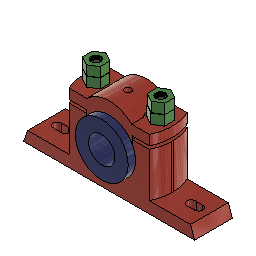
plumber block 3d (Autodesk Fusion 360 design; units mm, degrees)
Autodesk Fusion 360 part; units mm, degrees
sketch "Sketch1" plane through (0, 0, 0) normal (0, 1, 0) x (1, 0, 0)
  line L0 (23.6292, -4.2078) -> (27.987, -4.2078)
  line L1 (27.987, -4.2078) -> (27.987, -20.2078)
  line L2 (27.987, -20.2078) -> (53.987, -20.2078)
  line L3 (53.987, -20.2078) -> (53.987, 33.7922)
  line L4 (53.987, 33.7922) -> (98.9042, 33.7922)
  line L5 (103.9042, 47.7922) -> (-0.0958, 47.7922)
  line L6 (-0.0958, 47.7922) -> (-0.0958, 24.0008)
  line L7 (98.9042, 33.7922) -> (103.9042, 47.7922)
  arc A0 (23.6292, -4.2078) -> (-0.0958, 24.0008) centre (0, 0) ccw
  line L8 (-54.1786, 33.7922) -> (-99.0958, 33.7922)
  line L9 (-99.0958, 33.7922) -> (-104.0958, 47.7922)
  line L10 (-104.0958, 47.7922) -> (-0.0958, 47.7922)
  arc A1 (-0.0958, 24.0008) -> (-23.8208, -4.2078) centre (-0.1916, 0) ccw
  line L11 (-28.1786, -4.2078) -> (-28.1786, -20.2078)
  line L12 (-28.1786, -20.2078) -> (-54.1786, -20.2078)
  line L13 (-54.1786, -20.2078) -> (-54.1786, 33.7922)
  line L14 (-23.8208, -4.2078) -> (-28.1786, -4.2078)
  point P0 (-0.1916, 0)
  dimension "d3" = 26
  dimension "d5" = 16
  dimension "d6" = 104
  dimension "d7" = 5
  dimension "d39" = 68
  dimension "d61" = 44.9172
  dimension "d62" = 14
  constraint coincident A0.centre origin
  constraint perpendicular L0 L1
  constraint perpendicular L1 L2
  constraint perpendicular L2 L3
  constraint perpendicular L3 L4
  constraint perpendicular L5 L6
  constraint symmetric A0.centre L6 A1.centre
  constraint symmetric L0.end L6 L11.start
  constraint symmetric L1.end L6 L11.end
  constraint symmetric L2.end L6 L12.end
  constraint symmetric L3.end L6 L8.start
  constraint symmetric L4.end L6 L8.end
  constraint symmetric L5.start L6 L9.end
  constraint symmetric L5.end L6 L10.end
  constraint symmetric L6 A0.end A1.start
  constraint symmetric L6 L0.start A1.end
  constraint symmetric L6 A0 A1
  constraint horizontal L4
  constraint horizontal L5
  measures "d3" distance of L1.end L2.end
  measures "d5" distance of L0.end L1.end
  measures "d6" distance of L5.start L5.end
  measures "d7" horizontal distance of L4.end L5.start
  measures "d39" distance of L2.end L5
  measures "d61" distance of L3.end L4.end
  measures "d62" distance of L4 L5
extrude "Extrude1" add sketch "Sketch1" along normal mid plane 46 makes body 1
sketch "Sketch2" plane through (0, 0, 0) normal (0, 1, 0) x (1, 0, 0)
  line L0 (0, 0) -> (0, -8)
  line L1 (0, -8) -> (28, -8)
  line L2 (28, -8) -> (28, -24)
  line L3 (28, -24) -> (54, -24)
  line L4 (54, -24) -> (54, -36)
  line L5 (54, -36) -> (27.1477, -36)
  line L6 (-28, -24) -> (-54, -24)
  line L7 (-54, -36) -> (-27.1477, -36)
  line L8 (-28, -8) -> (-28, -24)
  line L9 (-54, -24) -> (-54, -36)
  line L10 (0, -8) -> (-28, -8)
  arc A0 (-22.6274, -8) -> (22.6274, -8) centre (0, 0) ccw
  arc A1 (-27.1477, -36) -> (27.1477, -36) centre (0, -8) ccw
  dimension "d11" = 8
  dimension "d12" = 28
  dimension "d13" = 16
  dimension "d14" = 26
  dimension "d15" = 12
  dimension "d64" = 48
  dimension "d65" = 78
  constraint coincident L0.start A0.centre
  constraint vertical L0
  constraint perpendicular L0 L1
  constraint perpendicular L1 L2
  constraint perpendicular L2 L3
  constraint perpendicular L1 L4
  constraint perpendicular L4 L5
  constraint coincident L1 A0.end
  constraint coincident L10 A0.start
  constraint coincident L0.end L1.start
  constraint horizontal L7
  measures "d11" distance of L0.start L0.end
  measures "d12" distance of L0.end L1.end
  measures "d13" distance of L1.end L2.end
  measures "d14" distance of L2.end L3.end
  measures "d15" distance of L3.end L4.end
  measures "d64" diameter of A0
  measures "d65" diameter of A1
extrude "Extrude2" add sketch "Sketch2" along normal mid plane 46 separate body contours L1 L2 L3 L4 L5 L6 L7 L8 L9 L10 A0 A1 makes body 2
sketch "Sketch3" plane through (0, 0, -47.7922) normal (0, 0, -1) x (1, 0, 0)
  line L0 (-104.0958, 23) -> (-104.0958, -23)
  line L1 (-104.0958, -23) -> (103.9042, -23)
  line L2 (103.9042, -23) -> (103.9042, 23)
  line L3 (103.9042, 23) -> (-104.0958, 23)
  circle A0 centre (0, 0) radius 4
  circle A1 centre (0, 0) radius 54
  circle A2 centre (0, 0) radius 83.1695
  circle A3 centre (38.9975, 0.4423) radius 7
  line L4 (51.9975, -12.5577) -> (25.9975, -12.5577)
  line L5 (25.9975, -12.5577) -> (25.9975, 13.4423)
  line L6 (25.9975, 13.4423) -> (51.9975, 13.4423)
  line L7 (51.9975, 13.4423) -> (51.9975, -12.5577)
  line L8 (51.9975, -12.5577) -> (25.9975, 13.4423) construction
  line L9 (25.9975, -12.5577) -> (51.9975, 13.4423) construction
  line L10 (0, 0) -> (-0.0958, 23)
  arc A4 (-78.3843, -5.3343) -> (-78.4652, 4.6223) centre (-77, -0.3444) ccw
  arc A5 (-86.4872, 4.5537) -> (-86.4043, -5.3996) centre (-86.4457, -0.4229) ccw
  line L11 (-51.8911, -12.9904) -> (-26.1085, 13.2253) construction
  line L12 (-25.892, -12.7738) -> (-52.1076, 13.0087) construction
  line L13 (-51.8911, -12.9904) -> (-25.892, -12.7738)
  line L14 (-78.3843, -5.3343) -> (-86.4043, -5.3996)
  line L15 (-86.4872, 4.5537) -> (-78.4652, 4.6223)
  line L16 (-25.892, -12.7738) -> (-26.1085, 13.2253)
  circle A6 centre (-38.9998, 0.1175) radius 7
  line L17 (-26.1085, 13.2253) -> (-52.1076, 13.0087)
  line L18 (-86.4457, -0.4229) -> (-77, -0.3444) construction
  line L19 (-52.1076, 13.0087) -> (-51.8911, -12.9904)
  line L20 (78.426, -4.6813) -> (86.4463, -4.6797)
  arc A7 (78.424, 5.2757) -> (78.426, -4.6813) centre (77.0002, 0.2969) ccw
  line L21 (86.4463, 0.2971) -> (77.0002, 0.2969) construction
  line L22 (86.4463, 5.2739) -> (78.424, 5.2757)
  arc A8 (86.4463, -4.6797) -> (86.4463, 5.2739) centre (86.4463, 0.2971) ccw
  point P0 (38.9975, 0.4423)
  point P1 (-38.9998, 0.1175)
  dimension "d20" = 8
  dimension "d21" = 108
  dimension "d22" = 14
  dimension "d23" = 26
  dimension "d24" = 26
  dimension "d27" = 39
  dimension "d63" = 77
  constraint coincident A0.centre A1.centre
  constraint concentric A0 A2
  constraint horizontal L4
  constraint perpendicular L4 L5
  constraint parallel L4 L6
  constraint parallel L5 L7
  constraint coincident L8 P0
  constraint coincident L9 P0
  constraint coincident P0 A3.centre
  constraint midpoint L3 L10.end
  constraint symmetric A3 L10 A6
  constraint symmetric L4.start L10 L11.start
  constraint symmetric L4.end L10 L12.start
  constraint symmetric L5.end L10 L11.end
  constraint symmetric L6.end L10 L12.end
  constraint symmetric P0 L10 P1
  constraint symmetric L10 A5.start L22.start
  constraint symmetric L10 A4.end A7.start
  constraint symmetric L10 A5.end L20.end
  constraint symmetric L10 A4.start L20.start
  constraint symmetric L10 A4 A7
  constraint symmetric L10 A5 A8
  measures "d20" diameter of A0
  measures "d21" diameter of A1
  measures "d22" diameter of A3
  measures "d23" distance of L5.end L6.end
  measures "d24" distance of L4.end L5.end
  measures "d27" distance of A0.centre P0
  measures "d63" horizontal distance of A0.centre A4.centre
extrude "Extrude3" cut sketch "Sketch3" against normal blind 80 from surface at -14 contours L1 L3 A1 A2 A4 L14 L15 | L1 L3 A1 A2 L20 A7 L22 | A2 A4 L14 L15 | A2 A5 L14 L15 bodies 1 2
extrude "Extrude4" cut sketch "Sketch3" against normal blind 120 contours A2 A4 L14 L15 | A2 A5 L14 L15 | A2 L20 L22 A8 | A2 L20 A7 L22 | A3 | A6 bodies 1 2
extrude "Extrude5" cut sketch "Sketch3" against normal blind 10 contours L4 L5 L6 L7 | L13 L16 L17 L19 bodies 1
extrude "Extrude8" cut sketch "Sketch3" against normal blind 25 contours A0 bodies 1
sketch "Sketch4" plane through (0, 0, 0) normal (1, 0, 0) x (0, 1, 0)
  line L0 (0, 0) -> (32, 0)
  line L1 (32, 0) -> (32, 32)
  line L2 (32, 32) -> (23, 32)
  line L3 (23, 32) -> (23, 24)
  line L4 (23, 24) -> (14, 24)
  line L5 (14, 24) -> (14, 22)
  line L6 (14, 22) -> (0, 22)
  line L7 (0, 22) -> (0, 0)
  line L8 (0, 16) -> (32, 16)
  line L9 (0, 0) -> (-32, 0)
  line L10 (0, 16) -> (-32, 16)
  line L11 (-14, 22) -> (0, 22)
  line L12 (-23, 32) -> (-23, 24)
  line L13 (-32, 32) -> (-23, 32)
  line L14 (-32, 0) -> (-32, 32)
  line L15 (-23, 24) -> (-14, 24)
  line L16 (-14, 24) -> (-14, 22)
  dimension "d43" = 32
  dimension "d44" = 32
  dimension "d45" = 23
  dimension "d46" = 14
  dimension "d47" = 24
  dimension "d48" = 22
  dimension "d49" = 16
  constraint coincident L0.start L7.end
  constraint horizontal L0
  constraint perpendicular L0 L1
  constraint perpendicular L1 L2
  constraint perpendicular L2 L3
  constraint perpendicular L3 L4
  constraint perpendicular L4 L5
  constraint perpendicular L5 L6
  constraint perpendicular L7 L8
  constraint symmetric L0.start L7 L9.start
  constraint symmetric L0.end L7 L9.end
  constraint symmetric L1.end L7 L13.start
  constraint symmetric L2.end L7 L12.start
  constraint symmetric L3.end L7 L12.end
  constraint symmetric L4.end L7 L15.end
  constraint symmetric L5.end L7 L11.start
  constraint symmetric L6.end L7 L11.end
  constraint symmetric L7 L8.end L10.end
  constraint midpoint L1 L8.end
  measures "d43" distance of L0.start L0.end
  measures "d44" distance of L0.end L1.end
  measures "d45" distance of L2.end L7
  measures "d46" distance of L5 L6.end
  measures "d47" distance of L0 L4
  measures "d48" distance of L0 L6
  measures "d49" vertical distance of L0.start L8.start
revolve "Revolve1" add sketch "Sketch4" angle 360 about axis through (0, 0, 0) along (0, 1, 0) separate body contours L7 L10 L11 L12 L13 L14 L15 L16 | L1 L2 L3 L4 L5 L6 L7 L8 makes body 3
extrude "Extrude7" add sketch "Sketch3" along normal blind 9 from surface at -27 contours A0 bodies 3
ref_plane "WorkPlane2" through (0, -5.0102, 47) normal (0, 0, 1) x (-1, 0, 0)
sketch "Sketch6" plane through (0, 0, 47) normal (0, 0, 1) x (1, 0, 0)
  circle A0 centre (0, 0) radius 4
  circle A1 centre (0, 0) radius 3
  dimension "d67" = 8
  dimension "d68" = 6
  constraint coincident A0.centre A1.centre
  measures "d67" diameter of A0
  measures "d68" diameter of A1
extrude "Extrude9" cut sketch "Sketch6" against normal blind 60 contours A1 bodies 2 3
extrude "Extrude10" cut sketch "Sketch6" against normal blind 16 bodies 2
sketch "Sketch7" plane through (0, 0, -37.7922) normal (0, 0, -1) x (1, 0, 0)
  circle A0 centre (-38.9998, 0.1175) radius 7
  line L0 (-52.1076, 13.0087) -> (-51.8911, -12.9904)
  line L1 (-51.8911, -12.9904) -> (-25.892, -12.7738)
  line L2 (-25.892, -12.7738) -> (-26.1085, 13.2253)
  line L3 (-26.1085, 13.2253) -> (-52.1076, 13.0087)
  circle A1 centre (-38.9998, 0.1175) radius 6
  line L4 (-26.9998, -11.8825) -> (-50.9998, -11.8825)
  line L5 (-50.9998, -11.8825) -> (-50.9998, 12.1175)
  line L6 (-50.9998, 12.1175) -> (-26.9998, 12.1175)
  line L7 (-26.9998, 12.1175) -> (-26.9998, -11.8825)
  line L8 (-26.9998, -11.8825) -> (-50.9998, 12.1175) construction
  line L9 (-50.9998, -11.8825) -> (-26.9998, 12.1175) construction
  point P0 (-38.9998, 0.1175)
  dimension "d75" = 12
  dimension "d76" = 24
  dimension "d77" = 24
  constraint concentric A0 A1
  constraint horizontal L4
  constraint perpendicular L4 L5
  constraint parallel L4 L6
  constraint parallel L5 L7
  constraint coincident L8 P0
  constraint coincident L9 P0
  constraint coincident P0 A0.centre
  measures "d75" diameter of A1
  measures "d76" distance of L5.end L6.end
  measures "d77" distance of L4.start L6.end
extrude "Extrude11" add sketch "Sketch7" along normal blind 8 separate body contours A0 | A1 | L4 L5 L6 L7 makes body 4
extrude "Extrude12" add sketch "Sketch7" against normal blind 95 contours A1 bodies 4
thread "Thread1" "ISO Metric profile 12.0 M12x1.75 6g" major diameter 11.8335 minor diameter 9.8365 pitch 1.75 angle 60 modelled right hand crest width 0.2518 on face at (-33.0073, 0.1816, 25.5412) from (-38.9998, -0.1175, 28.7078) to (-38.9998, -0.1175, 56.7078) crest through (-33.0831, -0.1175, -38.2297) on bodies 4
fillet "Fillet1" radius 8 curvature continuous 1 faces at (-42.9998, -4.1175, -45.7922) on bodies 4
sketch "Sketch8" plane through (0, 0, 36) normal (0, 0, 1) x (-1, 0, 0)
  circle A0 centre (38.9998, 0.1175) radius 7
  arc A1 (48.8569, -23) -> (48.8569, 23) centre (0, 0) ccw
  line L0 (48.8569, 23) -> (27.1477, 23)
  line L1 (27.1477, 23) -> (27.1477, -23)
  line L2 (27.1477, -23) -> (48.8569, -23)
  circle A2 centre (38.9998, 0.1175) radius 14.5
  circle A3 centre (38.9998, 0.1175) radius 6
  line L3 (28.6241, -6.155) -> (39.2441, -12.0044)
  line L4 (39.2441, -12.0044) -> (49.6198, -5.7319)
  line L5 (49.6198, -5.7319) -> (49.3755, 6.39)
  line L6 (49.3755, 6.39) -> (38.7555, 12.2394)
  line L7 (38.7555, 12.2394) -> (28.3798, 5.9669)
  line L8 (28.3798, 5.9669) -> (28.6241, -6.155)
  line L9 (0, 0) -> (0, -24.3708)
  circle A4 centre (-38.9998, 0.1175) radius 14.5
  circle A5 centre (-38.9998, 0.1175) radius 6
  circle A6 centre (-38.9998, 0.1175) radius 7
  line L10 (-28.3798, 5.9669) -> (-28.6241, -6.155)
  circle A7 centre (-38.9998, 0.1175) radius 6
  line L11 (-28.6241, -6.155) -> (-39.2441, -12.0044)
  line L12 (-38.7555, 12.2394) -> (-28.3798, 5.9669)
  line L13 (-49.6198, -5.7319) -> (-49.3755, 6.39)
  line L14 (-49.3755, 6.39) -> (-38.7555, 12.2394)
  line L15 (-39.2441, -12.0044) -> (-49.6198, -5.7319)
  point P0 (38.9998, 0.1175)
  point P1 (-38.9998, 0.1175)
  point P2 (-38.9998, 0.1175)
  dimension "d86" = 29
  dimension "d87" = 12
  dimension "d88" = 10.5
  constraint concentric A0 A2
  constraint concentric A0 A3
  constraint coincident P0 A0.centre
  constraint coincident A1.centre L9.start
  constraint vertical L9
  constraint symmetric A2 L9 A4
  constraint symmetric A3 L9 A5
  constraint symmetric A0 L9 A6
  constraint symmetric P0 L9 P2
  constraint symmetric A3 L9 A7
  constraint symmetric L3.start L9 L10.end
  constraint symmetric L3.end L9 L11.end
  constraint symmetric L4.end L9 L13.start
  constraint symmetric L5.end L9 L13.end
  constraint symmetric L6.end L9 L12.start
  constraint symmetric L7.end L9 L10.start
  measures "d86" diameter of A2
  measures "d87" diameter of A3
  measures "d88" distance of P0 L8
extrude "Extrude13" cut sketch "Sketch8" along normal blind 30 contours L1 A2 | A4 | A6 | L10 L11 L12 L13 L14 L15 picked at (26.8057, -2.1038) bodies 2
extrude "Extrude14" add sketch "Sketch8" along normal blind 12 separate body contours A0 | L3 L4 L5 L6 L7 L8 makes body 5
ref_plane "WorkPlane3" through (-49.3755, -6.39, 36) normal (-0.48245, -0.875924, 0) x (0.875924, -0.48245, 0)
copy_body "CopyPasteBodies1" bodies 4 makes body 6
move_body "Move1" bodies 6 to x (1, 0, 0) y (0, 1, 0) z (0, 0, 1) at (160, 0, 0)
copy_body "Body->Comp1" bodies 1 removing the originals makes body 7 in component "Component"
copy_body "Body->Comp2" bodies 2 removing the originals makes body 8 in component "Component'"
copy_body "Body->Comp3" bodies 3 removing the originals makes body 9 in component "Component''"
copy_body "Body->Comp4" bodies 4 removing the originals makes body 10 in component "Component'''"
copy_body "Body->Comp5" bodies 5 removing the originals makes body 11 in component "Component''''"
copy_body "Body->Comp7" bodies 6 removing the originals makes body 12 in component "Component'''''"
thread "Thread1'" "ISO Metric profile 12.0 M12x1.5 6H" major diameter 12.203 minor diameter 10.526 pitch 1.5 angle 60 modelled right hand crest width 0.4065 on face at (-44.9924, 0.1816, 44) crest through (-44.2628, -0.1175, 36.375) on bodies 11 in component "Component''''"
copy_body "CopyPasteBodies2" bodies 11 makes body 13
move_body "Move2" bodies 13 to x (1, 0, 0) y (0, 1, 0) z (0, 0, 1) at (-34.4957, 26.1177, 25.0582)
copy_body "Body->Comp8" bodies 13 removing the originals makes body 14 in component "Component''''''"
copy_body "CopyPasteBodies3" bodies 11 makes body 15
move_body "Move3" bodies 15 to x (1, 0, 0) y (0, 1, 0) z (0, 0, 1) at (0, 0, 15)
copy_body "CopyPasteBodies4" bodies 14 makes body 16
move_body "Move4" bodies 16 to x (1, 0, 0) y (0, 1, 0) z (0, 0, 1) at (0, 0, 20)
copy_body "Body->Comp9" bodies 16 removing the originals makes body 17 in component "Component'''''''"
copy_body "Body->Comp10" bodies 15 removing the originals makes body 18 in component "Component''''''''"
component "Component" placed x (1, 0, 0) y (0, 1, 0) z (0, 0, 1) at (0, 0, 0)
component "Component'" placed x (1, 0, 0) y (0, 1, 0) z (0, 0, 1) at (0, 0, 0)
component "Component''" placed x (1, 0, 0) y (0, 1, 0) z (0, 0, 1) at (0, 0, 0)
component "Component'''" placed x (1, 0, 0) y (0, 1, 0) z (0, 0, 1) at (0, 0, -1.2078)
component "Component''''" placed x (1, 0, 0) y (0, 1, 0) z (0, 0, 1) at (0, 0, 0)
component "Component'''''" placed x (1, 0, 0) y (0, 1, 0) z (0, 0, 1) at (-82.0004, 0, -1.2078)
component "Component''''''" placed x (1, 0, 0) y (0, 1, 0) z (0, 0, 1) at (0, 0, 0)
component "Component'''''''" placed x (1, 0, 0) y (0, 1, 0) z (0, 0, 1) at (0, 0, 0)
component "Component''''''''" placed x (1, 0, 0) y (0, 1, 0) z (0, 0, 1) at (0, 0, 0)
